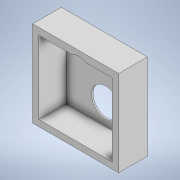
# Autodesk Inventor part: ledbox
Saved by Autodesk Inventor 2022 (Build 260153000, 153)
## iProperties
Created: 2021-07-02
Part Number: ledbox
Material: Generic
Document SubType Name: Modeling
Designer: 91852
Density: 1 g/cm^3
Appearance: Default
Author: 91852
Autodesk Inventor part; units mm, degrees
ref_plane "YZ Plane" through (0, 0, 0) normal (1, 0, 0) x (0, 1, 0)
ref_plane "XZ Plane" through (0, 0, 0) normal (0, 1, 0) x (-1, 0, 0)
ref_plane "XY Plane" through (0, 0, 0) normal (0, 0, 1) x (1, 0, 0)
sketch "Sketch1" plane through (0, 0, 0) normal (0, 0, 1) x (1, 0, 0)
  line L0 (-15.4228, 9.2021) -> (98.8772, 9.2021)
  line L1 (98.8772, 9.2021) -> (98.8772, -105.0979)
  line L2 (98.8772, -105.0979) -> (-15.4228, -105.0979)
  line L3 (-15.4228, -105.0979) -> (-15.4228, 9.2021)
  point P0 (0, 0)
  dimension "d0" = 114.3
  dimension "d1" = 114.3
  constraints: 8 end point, 2 parallel, 1 horizontal, 1 perpendicular
  measures "d0" distance of L1.end L2.end
  measures "d1" distance of L0.end L1.end
extrude "Extrusion1" add sketch "Sketch1" along normal blind 38.1
sketch "Sketch2" plane through (0, 0, 38.1) normal (0, 0, 1) x (1, 0, 0)
  line L0 (-6.9895, 0) -> (90.3039, 0)
  line L1 (90.3039, 0) -> (90.3039, -96.7342)
  line L2 (90.3039, -96.7342) -> (-6.9895, -96.7342)
  line L3 (-6.9895, -96.7342) -> (-6.9895, 0)
  point P0 (0, 0)
  constraints: 8 end point, 2 parallel, 1 horizontal, 1 perpendicular
extrude "Extrusion2" cut sketch "Sketch2" against normal blind 36
sketch "Sketch3" plane through (0, 0, 0) normal (0, 0, -1) x (-1, 0, 0)
  circle A0 centre (-45.7039, -16.5922) radius 19.05
  circle A1 centre (-45.7039, -68.7821) radius 19.05
  point P0 (0, 0)
  dimension "d6" = 38.1
  dimension "d7" = 38.1
  constraints: 2 centre point
  measures "d6" diameter of A0
  measures "d7" diameter of A1
extrude "Extrusion3" cut sketch "Sketch3" against normal through all
body "Solid1"
